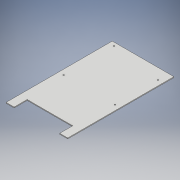
# Autodesk Inventor part: trunk
Saved by Autodesk Inventor 2018 (Build 220112000, 112)
## iProperties
Created: 2018-06-06
Part Number: trunk
Material: Generic
Document SubType Name: Modeling
Designer: John Viljoen
Density: 1 g/cm^3
Appearance: Default
Author: John Viljoen
Autodesk Inventor part; units mm, degrees
ref_plane "YZ Plane" through (0, 0, 0) normal (1, 0, 0) x (0, 1, 0)
ref_plane "XZ Plane" through (0, 0, 0) normal (0, 1, 0) x (-1, 0, 0)
ref_plane "XY Plane" through (0, 0, 0) normal (0, 0, 1) x (1, 0, 0)
sketch "Sketch1" plane through (0, 0, 0) normal (0, 0, 1) x (1, 0, 0)
  line L0 (0, 0) -> (189.177, 0)
  line L1 (189.177, 0) -> (189.177, 325.825)
  line L2 (189.177, 325.825) -> (0, 325.825)
  line L3 (0, 325.825) -> (0, 0)
  dimension "d0" = 189.177
  dimension "d1" = 325.825
  constraints: 8 end point, 2 parallel, 1 horizontal, 1 perpendicular
  measures "d0" distance of L2.end L1.end
  measures "d1" distance of L1.end L0.end
extrude "Extrusion1" add sketch "Sketch1" along normal blind 2.6
sketch "Sketch2" plane through (0, 0, 2.6) normal (0, 0, 1) x (1, 0, 0)
  line L0 (0, 325.825) -> (0, 0) projected
  line L1 (0, 170) -> (0, 0)
  line L2 (0, 170) -> (0, 159.84) construction
  line L3 (0, 159.84) -> (6.35, 159.84) construction
  line L4 (6.35, 170) -> (163.83, 170) construction
  line L5 (163.83, 170) -> (163.83, 136.98) construction
  line L6 (6.35, 159.84) -> (6.35, 4.9) construction
  line L7 (6.35, 4.9) -> (163.83, 4.9) construction
  line L8 (6.35, 159.84) -> (15.9385, 159.84) construction
  line L9 (15.9385, 159.84) -> (15.9385, 4.9) construction
  line L10 (163.83, 136.98) -> (173.4185, 136.98) construction
  line L11 (173.4185, 136.98) -> (173.4185, 4.9) construction
  line L12 (0, 325.825) -> (0, 315.665) construction
  line L13 (15.9385, 159.84) -> (15.9385, 315.665) construction
  line L14 (173.4185, 136.98) -> (173.4185, 292.805) construction
  line L15 (15.9385, 4.9) -> (15.9385, 160.725) construction
  line L16 (173.4185, 4.9) -> (173.4185, 160.725) construction
  circle A0 centre (173.4185, 160.725) radius 1.98
  circle A1 centre (15.9385, 160.725) radius 1.98
  circle A2 centre (15.9385, 315.665) radius 1.98
  circle A3 centre (173.4185, 292.805) radius 1.98
  dimension "d4" = 10.16
  dimension "d6" = 157.48
  dimension "d7" = 33.02
  dimension "d8" = 154.94
  dimension "d13" = 9.5885
  dimension "d14" = 9.5885
  dimension "d19" = 10.16
  dimension "d20" = 155.825
  dimension "d21" = 155.825
  dimension "d22" = 155.825
  dimension "d23" = 3.96
  dimension "d24" = 3.96
  dimension "d25" = 3.96
  dimension "d26" = 3.96
  constraints: 32 end point, 10 coincident, 6 point on line, 5 perpendicular, 4 centre point, 2 horizontal, 2 vertical
  measures "d4" distance of L1.start L2.end
  measures "d6" distance of L4.start L4.end
  measures "d7" distance of L4.end L5.end
  measures "d8" distance of L3.end L6.end
  measures "d13" distance of L8.start L8.end
  measures "d14" distance of L10.start L10.end
  measures "d19" distance of L0.start L12.end
  measures "d20" distance of L14.start L14.end
  measures "d21" distance of L15.start L15.end
  measures "d22" distance of L16.start L16.end
  measures "d23" diameter of A0
  measures "d24" diameter of A1
  measures "d25" diameter of A2
  measures "d26" diameter of A3
extrude "Extrusion2" cut sketch "Sketch2" against normal blind 5
sketch "Sketch4" plane through (0, 0, 2.6) normal (0, 0, 1) x (1, 0, 0)
  line L0 (0, 0) -> (189.177, 0) projected
  line L1 (189.177, 0) -> (164.5885, 0) construction
  line L2 (164.5885, 0) -> (24.5885, 0)
  line L3 (24.5885, 0) -> (24.5885, 40)
  line L4 (24.5885, 40) -> (164.5885, 40)
  line L5 (164.5885, 40) -> (164.5885, 0)
  dimension "d29" = 24.5885
  dimension "d30" = 140
  dimension "d31" = 40
  constraints: 10 end point, 2 parallel, 1 horizontal, 1 perpendicular, 1 point on line
  measures "d29" distance of L0.end L1.end
  measures "d30" distance of L3.end L4.end
  measures "d31" distance of L2.end L3.end
extrude "Extrusion3" cut sketch "Sketch4" against normal blind 10
body "Solid1"
